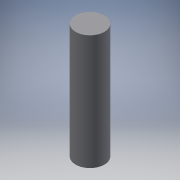
# Autodesk Inventor part: cilindro_tal
Saved by Autodesk Inventor 2018 (Build 220112000, 112)
## iProperties
Created: 2021-07-10
Part Number: cilindro_tal
Material: Genérico
Document SubType Name: Modeling
Designer: GABRIEL
Density: 1 g/cm^3
Appearance: Valor por defecto
Author: GABRIEL
Autodesk Inventor part; units mm, degrees
ref_plane "YZ Plane" through (0, 0, 0) normal (1, 0, 0) x (0, 1, 0)
ref_plane "XZ Plane" through (0, 0, 0) normal (0, 1, 0) x (-1, 0, 0)
ref_plane "XY Plane" through (0, 0, 0) normal (0, 0, 1) x (1, 0, 0)
sketch "Boceto1" plane through (0, 0, 0) normal (0, 0, 1) x (1, 0, 0)
  circle A0 centre (0, 0) radius 12.5
  dimension "d0" = 25
  constraints: 1 centre point, 1 coincident
  measures "d0" diameter of A0
extrude "Extrusión1" add sketch "Boceto1" along normal blind 180
